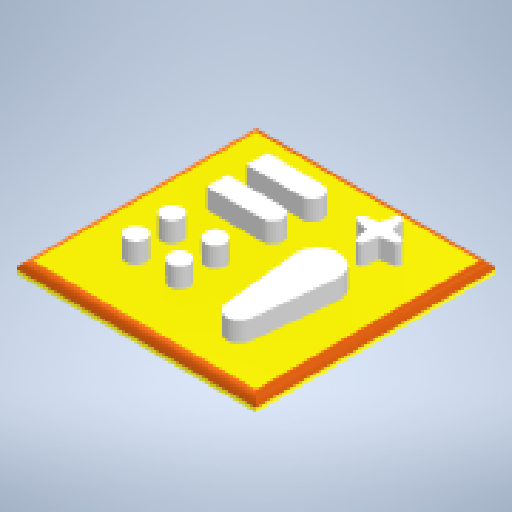
# Autodesk Inventor part: Lamina
Saved by Autodesk Inventor 2025.2 (Build 292293000, 293)
## iProperties
Created: 2025-02-17
Part Number: Lamina
Material: Genérico
Document SubType Name: Modeling
Designer: hmont
Density: 1 g/cm^3
Appearance: Valor por defecto
Author: hmont
Autodesk Inventor part; units mm, degrees
ref_plane "YZ Plane" through (0, 0, 0) normal (1, 0, 0) x (0, 1, 0)
ref_plane "XZ Plane" through (0, 0, 0) normal (0, 1, 0) x (-1, 0, 0)
ref_plane "XY Plane" through (0, 0, 0) normal (0, 0, 1) x (1, 0, 0)
sketch "Boceto1" plane through (0, 0, 0) normal (0, 1, 0) x (-1, 0, 0)
  line L0 (0, 0) -> (600, 0)
  line L1 (600, 0) -> (600, -600)
  line L2 (600, -600) -> (0, -600)
  line L3 (0, -600) -> (0, 0)
  dimension "d0" = 600
  dimension "d1" = 600
  constraints: 8 end point, 2 parallel, 1 horizontal, 1 perpendicular
  measures "d0" distance of L0.end L1.end
  measures "d1" distance of L1.end L2.end
extrude "Extrusión1" add sketch "Boceto1" along normal blind 30
fillet "Empalme1" radius 20 4 edges at (-300, 30, 0) (0, 30, -300) (-300, 30, -600) (-600, 30, -300)
sketch "Boceto2" plane through (0, 30, 0) normal (0, 1, 0) x (1, 0, 0)
  circle A0 centre (-350.7134, 158.3807) radius 25
  circle A1 centre (-459.5461, 158.3807) radius 25
  circle A2 centre (-350.7134, 248.7418) radius 25
  circle A3 centre (-459.5461, 248.7418) radius 25
  arc A4 (-195.2633, 121.4375) -> (-130.7405, 121.4375) centre (-163.0019, 121.4375) ccw
  arc A5 (-110.2556, 305.231) -> (-215.7481, 305.231) centre (-163.0019, 317.1367) ccw
  line L0 (-108.9286, 317.1367) -> (-130.7405, 121.4375)
  line L1 (-195.2633, 121.4375) -> (-217.0751, 317.1367)
  arc A6 (-333.7394, 348.6874) -> (-333.7394, 401.4079) centre (-333.7394, 375.0477) ccw
  line L2 (-333.7394, 348.6874) -> (-472.5261, 348.6874)
  line L3 (-333.7394, 401.4079) -> (-472.5261, 401.4079)
  line L4 (-472.5261, 401.4079) -> (-472.5261, 348.6874)
  arc A7 (-331.4434, 446.537) -> (-331.4434, 499.2575) centre (-331.4434, 472.8973) ccw
  line L5 (-331.4434, 446.537) -> (-470.23, 446.537)
  line L6 (-331.4434, 499.2575) -> (-470.23, 499.2575)
  line L7 (-470.23, 499.2575) -> (-470.23, 446.537)
  circle A8 centre (-163.585, 428.2615) radius 10.0613
  circle A9 centre (-118.3661, 472.3141) radius 10.0613
  circle A10 centre (-162.4187, 517.5331) radius 10.0613
  circle A11 centre (-207.6377, 473.4804) radius 10.0613
  line L8 (-118.2811, 462.2532) -> (-147.5182, 456.7387)
  line L9 (-118.3661, 482.3754) -> (-147.0901, 488.3237)
  line L10 (-152.3603, 517.7711) -> (-147.0901, 488.3237)
  line L11 (-172.48, 517.5331) -> (-178.4251, 488.9079)
  line L12 (-208.7596, 483.4789) -> (-178.4251, 488.9079)
  line L13 (-173.6463, 428.2615) -> (-178.9246, 457.3337)
  line L14 (-208.529, 463.4587) -> (-178.9246, 457.3337)
  line L15 (-153.5449, 427.6096) -> (-147.5182, 456.7387)
  point P0 (0, 0)
  point P1 (-163.0019, 472.8973)
  point P2 (-163.0019, 472.8973)
  point P3 (-163.0019, 472.8973)
  point P4 (-163.0019, 472.8973)
  dimension "d5" = 50
  dimension "d6" = 50
  dimension "d7" = 50
  dimension "d8" = 50
  dimension "d11" = 360
  constraints: 32 end point, 18 point on circle, 12 centre point, 2 coincident, 2 horizontal, 2 perpendicular, 2 point on line, 2 tangent, 2 vertical, 11 other
  measures "d5" diameter of A0
  measures "d6" diameter of A1
  measures "d7" diameter of A2
  measures "d8" diameter of A3
extrude "Extrusión2" add sketch "Boceto2" along normal blind 50 contours A0 | A1 | A2 | A3 | L1 A5 L0 A4 | L2 L4 L3 A6 | L5 L7 L6 A7 | A8 | A8 L13 L14 A11 L12 L11 A10 L10 L9 A9 L8 L15 | A11 | A9 | A10
